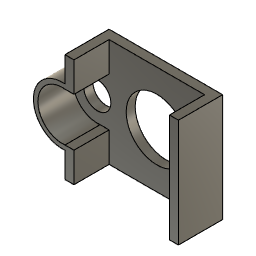
power_button_holder (Autodesk Fusion 360 design; units mm, degrees)
Autodesk Fusion 360 part; units mm, degrees
sketch "Sketch1" plane through (0, 0, 0) normal (0, 1, 0) x (1, 0, 0)
  circle A0 centre (24.3, -25) radius 3.4
  circle A1 centre (24.3, -25) radius 3.5
  line L0 (20.2, -31) -> (28.4, -31)
  line L1 (28.4, -31) -> (28.4, -19)
  line L2 (28.4, -19) -> (20.2, -19)
  line L3 (20.2, -19) -> (20.2, -31)
  line L4 (16.3899, -35.3633) -> (33, -35.3633)
  line L5 (33, -35.3633) -> (33, -15)
  line L6 (33, -15) -> (16.3899, -15)
  line L7 (16.3899, -15) -> (16.3899, -35.3633)
  line L8 (20.2, -31) -> (19.2, -31)
  line L9 (19.2, -31) -> (19.2, -19)
  line L10 (19.2, -19) -> (20.2, -19)
  line L11 (20.2, -19) -> (20.2, -31)
  line L12 (28.4, -31) -> (29.4, -31)
  line L13 (29.4, -31) -> (29.4, -19)
  line L14 (29.4, -19) -> (28.4, -19)
  line L15 (28.4, -19) -> (28.4, -31)
  circle A2 centre (17.7, -25) radius 1.5
  circle A3 centre (17.7, -25) radius 2.5
  line L16 (17.7, -27.5) -> (19.2, -27.5)
  line L17 (17.7, -22.5) -> (19.2, -22.5)
  circle A4 centre (17.7, -25) radius 2.7
  circle A5 centre (17.7, -25) radius 3.2
  line L18 (18, -31) -> (19, -31)
  line L19 (19, -31) -> (19, -27.924)
  line L20 (19, -27.924) -> (18, -27.924)
  line L21 (18, -27.924) -> (18, -31)
  line L22 (19, -22.076) -> (18, -22.076)
  line L23 (18, -22.076) -> (18, -19)
  line L24 (18, -19) -> (19, -19)
  line L25 (19, -19) -> (19, -22.076)
  line L26 (29.6, -31) -> (30.6, -31)
  line L27 (30.6, -31) -> (30.6, -19)
  line L28 (30.6, -19) -> (29.6, -19)
  line L29 (29.6, -19) -> (29.6, -31)
  line L30 (30.6, -31) -> (18, -31)
  line L31 (18, -31) -> (18, -19)
  line L32 (18, -19) -> (30.6, -19)
  line L33 (30.6, -19) -> (30.6, -31)
  line L34 (18, -27.6833) -> (19, -27.6833)
  line L35 (19, -27.6833) -> (19, -27.924)
  line L36 (19, -27.924) -> (18, -27.924)
  line L37 (18, -27.924) -> (18, -27.6833)
  line L38 (18, -22.3167) -> (19, -22.3167)
  line L39 (19, -22.3167) -> (19, -22.076)
  line L40 (19, -22.076) -> (18, -22.076)
  line L41 (18, -22.076) -> (18, -22.3167)
  dimension "d1" = 6.8
  dimension "d2" = 7
  dimension "d3" = 8.2
  dimension "d4" = 12
  dimension "d5" = 4.1
  dimension "d6" = 6
  dimension "d7" = 1
  dimension "d8" = 12
  dimension "d9" = 1
  dimension "d10" = 12
  dimension "d15" = 3
  dimension "d16" = 5
  dimension "d17" = 1.5
  dimension "d22" = 5.4
  dimension "d23" = 6.4
  dimension "d24" = 1
  dimension "d25" = 0.2
  dimension "d26" = 0.2
  dimension "d27" = 1
  dimension "d28" = 0.2
  dimension "d29" = 1
  constraint concentric A0 A1
  constraint horizontal L0
  constraint vertical L1
  constraint horizontal L2
  constraint vertical L3
  constraint horizontal L4
  constraint vertical L5
  constraint horizontal L6
  constraint vertical L7
  constraint horizontal L8
  constraint vertical L9
  constraint horizontal L10
  constraint vertical L11
  constraint horizontal L12
  constraint vertical L13
  constraint horizontal L14
  constraint vertical L15
  constraint concentric A2 A3
  constraint coincident A3 L16.start
  constraint coincident L9 L16.end
  constraint tangent A3 L16
  constraint perpendicular L9 L16
  constraint coincident A3 L17.start
  constraint coincident L9 L17.end
  constraint tangent A3 L17
  constraint perpendicular L9 L17
  constraint concentric A2 A4
  constraint concentric A4 A5
  constraint horizontal L18
  constraint vertical L19
  constraint horizontal L20
  constraint vertical L21
  constraint coincident A5 L19.end
  constraint horizontal L22
  constraint vertical L23
  constraint horizontal L24
  constraint vertical L25
  constraint coincident A5 L22.start
  constraint horizontal L26
  constraint vertical L27
  constraint horizontal L28
  constraint vertical L29
  constraint horizontal L30
  constraint vertical L31
  constraint horizontal L32
  constraint vertical L33
  constraint horizontal L34
  constraint vertical L35
  constraint horizontal L36
  constraint vertical L37
  constraint coincident L31 L34.start
  constraint coincident A4 L34.start
  constraint horizontal L38
  constraint vertical L39
  constraint horizontal L40
  constraint vertical L41
  constraint coincident A4 L38.start
  constraint coincident L31 L38.start
  measures "d1" diameter of A0
  measures "d2" diameter of A1
  measures "d3" distance of L0.start L0.end
  measures "d4" distance of L0.start L2.end
  measures "d5" distance of A0.centre L3
  measures "d6" distance of A0.centre L2
  measures "d7" distance of L0.start L8.end
  measures "d8" distance of L0.start L2.end
  measures "d9" distance of L0.end L12.end
  measures "d10" distance of L0.end L1.end
  measures "d15" diameter of A2
  measures "d16" diameter of A3
  measures "d17" distance of L9 A2.centre
  measures "d22" diameter of A4
  measures "d23" diameter of A5
  measures "d24" distance of L18.start L18.end
  measures "d25" distance of L9 L19
  measures "d26" distance of L9 L25
  measures "d27" distance of L23.end L24.end
  measures "d28" distance of L13 L29
  measures "d29" distance of L26.start L26.end
extrude "Extrude1" add sketch "Sketch1" along normal blind 2 contours A1 L0 L1 L2 L3 L11 L15 A5 L30 L32 | A1 L3 L11 A4 A5 | L3 L9 L10 L11 A5 L32 | L3 L9 L11 A4 A5 | L3 L9 L11 A4 A5 | L3 L8 L9 L11 A5 L30 | L3 L11 A4 | L3 L9 L11 A3 A4 | L3 L9 L11 A3 A4 | L1 L12 L13 L14 L15 L30 L32 | L9 A3 makes body 1
extrude "Extrude2" add sketch "Sketch1" against normal blind 3.9 contours L3 L9 L10 L11 A5 L32 | L3 L9 L11 A4 A5 | L3 L9 L11 A4 A5 | L3 L8 L9 L11 A5 L30 | L3 L9 L11 A3 A4 | L3 L9 L11 A3 A4 | L1 L12 L13 L14 L15 L30 L32 | L9 A3 bodies 1
extrude "Extrude3" add sketch "Sketch1" along normal blind 2 contours L9 L17 A4 | L9 A3 L17 A4 L31 | L9 A3 L16 A4 L31 | L9 L16 A4 | L9 A2 A3 L31 | L9 A2 A3 L31 | A2 L31 | L7 A2 A3 L31 | A3 L17 L31 | A3 L16 L31 | L7 A2 A3 L31 | L7 A2 L31 | L7 A2 A3 | L7 A2 bodies 1
extrude "Extrude4" add sketch "Sketch1" against normal blind 3.9 contours L9 L17 A4 | L9 A3 L17 A4 L31 | L9 A3 L16 A4 L31 | L9 L16 A4 | L9 A2 A3 L31 | L9 A2 A3 L31 | L7 A2 A3 L31 | A3 L17 L31 | A3 L16 L31 | L7 A2 A3 L31 | L7 A2 A3 bodies 1
extrude "Extrude5" add sketch "Sketch1" along normal blind 1 separate body contours A1 A5 | A1 A5 | A1 L0 L1 L2 L3 L11 L15 A5 L30 L32 | A1 L3 L11 A4 A5 | L3 L9 L10 L11 A5 L32 | L3 L9 L11 A4 A5 | L3 L9 L11 A4 A5 | L3 L8 L9 L11 A5 L30 | L3 L11 A4 | L3 L9 L11 A3 A4 | L9 A5 L25 L32 | L9 L17 A4 A5 L38 L39 | L3 L9 L11 A3 A4 | L9 L16 A4 A5 L34 L35 | L9 A5 L19 L30 | L1 L12 L13 L14 L15 L30 L32 | L9 A3 | L9 L17 A4 | L9 A3 L17 A4 L31 | A5 L22 L23 L31 L40 | L22 L31 L38 L39 L40 L41 | A5 L23 L24 L25 L31 L32 | L9 A3 L16 A4 L31 | L9 L16 A4 | A5 L18 L19 L21 L30 L31 | A5 L20 L21 L31 L36 | L20 L31 L34 L35 L36 L37 | L13 L29 L30 L32 | L9 A2 A3 L31 | L9 A2 A3 L31 | L17 A4 L31 | L7 A4 A5 L23 L31 L41 | L16 A4 L31 | L7 A4 A5 L21 L31 L37 | L26 L27 L28 L29 L30 L32 L33 | A2 L31 | L7 A2 A3 L31 | A3 L17 L31 | A3 L16 L31 | L7 A2 A3 L31 | L7 A3 L17 A4 L31 | L7 A4 A5 | L7 A3 L16 A4 L31 | L7 A2 L31 | L7 A3 A4 | L7 A2 A3 | L7 A2 makes body 2
extrude "Extrude6" add sketch "Sketch1" against normal blind 3.9 contours A5 L22 L23 L31 L40 | L22 L31 L38 L39 L40 L41 | A5 L23 L24 L25 L31 L32 | A5 L18 L19 L21 L30 L31 | A5 L20 L21 L31 L36 | L20 L31 L34 L35 L36 L37 | L7 A4 A5 L23 L31 L41 | L7 A4 A5 L21 L31 L37 | L26 L27 L28 L29 L30 L32 L33 | L7 A4 A5 bodies 2
extrude "Extrude7" cut sketch "Sketch1" along normal blind 2 contours A2 L31 | L7 A2 L31 | L7 A2 bodies 2
hidden bodies 1
